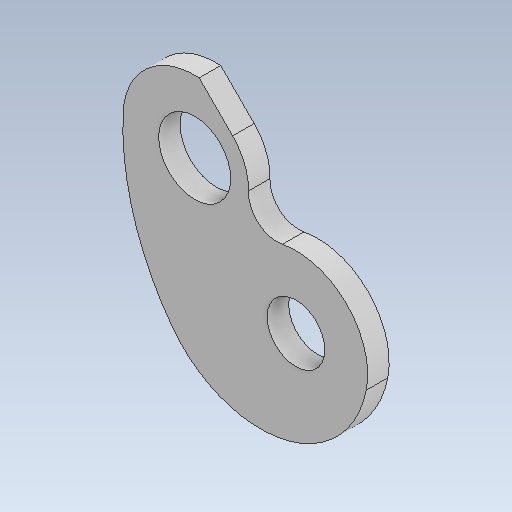
# Autodesk Inventor part: 従動節
Saved by Autodesk Inventor 2020.4 (Build 244396000, 396)
## iProperties
Created: 2021-05-01
Part Number: 従動節
Material: 一般
Document SubType Name: Modeling
Designer: happy
Density: 1 g/cm^3
Appearance: 既定
Mass: 2.14193 g
Surface Area: 19.4138 cm^2
Volume: 2.14193 cm^3
Author: happy
Autodesk Inventor part; units mm, degrees
ref_plane "YZ Plane" through (0, 0, 0) normal (1, 0, 0) x (0, 1, 0)
ref_plane "XZ Plane" through (0, 0, 0) normal (0, 1, 0) x (-1, 0, 0)
ref_plane "XY Plane" through (0, 0, 0) normal (0, 0, 1) x (1, 0, 0)
sketch "スケッチ1" plane through (0, 0, 0) normal (0, 0, 1) x (1, 0, 0)
  circle A0 centre (0, 0) radius 5.025
  circle A1 centre (0, 0) radius 10
  line L0 (0, 0) -> (14.1421, -14.1421)
  line L1 (0, 0) -> (20, 0) construction
  line L2 (0, 0) -> (14.1421, -14.1421) construction
  line L3 (-7.0711, -7.0711) -> (7.0711, -21.2132)
  line L4 (21.2132, -7.0711) -> (7.0711, 7.0711)
  arc A2 (7.0711, 7.0711) -> (-7.0711, -7.0711) centre (0, 0) ccw
  arc A3 (7.0711, -21.2132) -> (21.2132, -7.0711) centre (14.1421, -14.1421) ccw
  circle A4 centre (14.1421, -14.1421) radius 4.025
  circle A5 centre (14.1421, -14.1421) radius 13
  circle A6 centre (14.1421, -14.1421) radius 14
  line L5 (4.2426, -24.0416) -> (21.0227, -40.8217)
  line L6 (21.0227, -40.8217) -> (47.0109, -27.2119)
  line L7 (47.0109, -27.2119) -> (24.0416, -4.2426)
  arc A7 (12.0122, -27.9792) -> (10.7234, -30.5224) centre (11.784, -29.4617) ccw
  line L8 (-8.3867, -5.4464) -> (8.8712, -32.0212)
  arc A8 (10.5855, -29.4018) -> (10.585, -29.4134) centre (11.784, -29.4617) ccw
  line L9 (4.2426, -24.0416) -> (21.0227, -40.8217)
  line L10 (21.0227, -40.8217) -> (47.0109, -27.2119)
  line L11 (47.0109, -27.2119) -> (24.0416, -4.2426)
  arc A9 (8.8712, -32.0212) -> (10.7228, -30.5218) centre (9.8758, -31.3688) ccw
  arc A10 (11.5527, -27.9797) -> (10.7228, -30.5218) centre (11.784, -29.4617) ccw
  arc A11 (11.5527, -27.9797) -> (23.9469, -16.1083) centre (9.2397, -13.1591) ccw
  arc A12 (-9.9898, 0.4505) -> (9.3407, -32.4405) centre (24.9746, -1.1263) ccw
  arc A13 (21.2132, -7.0711) -> (7.0711, -21.2132) centre (14.1421, -14.1421) ccw
  arc A14 (7.4956, -0.2576) -> (12.25, -4.3228) centre (11.4932, -0.395) ccw
  circle A15 centre (0, 0) radius 7.5
  line L12 (5.3033, 5.3033) -> (0.6262, 9.9804)
  arc A16 (-3.1585, -21.9475) -> (11.5527, -27.9797) centre (9.1773, -12.8178) ccw
  point P0 (7.0711, -7.0711)
  point P1 (7.0711, 7.0711)
  point P2 (10.4941, -23.453)
  point P3 (-8.3867, -5.4464)
  point P4 (9.5568, -27.6782)
  point P5 (9.5574, -27.6666)
  point P6 (-9.9898, 0.4505)
  point P7 (10.7234, -30.5224)
  point P8 (11.5527, -27.9797)
  point P9 (9.2796, -3.7267)
  point P10 (0.6262, 9.9804)
  dimension "d0" = 10.05
  dimension "d1" = 20
  dimension "d2" = 20
  dimension "d3" = 45
  dimension "d6" = 8.05
  dimension "d7" = 26
  dimension "d8" = 1
  dimension "d9" = 1.5
  dimension "d14" = 0
  dimension "d15" = 0
  dimension "d17" = 15
  dimension "d18" = 168
  dimension "d19" = 35
  dimension "d20" = 4
  dimension "d21" = 15
  constraints: 35 point on circle, 28 end point, 22 tangent, 17 centre point, 5 coincident, 4 parallel, 2 point on line, 1 collinear, 1 equal length, 1 horizontal, 1 midpoint, 2 other
  measures "d0" diameter of A0
  measures "d1" diameter of A1
  measures "d2" distance of L0.start L0.end
  measures "d3" angle of L0 L1
  measures "d6" diameter of A4
  measures "d7" diameter of A5
  measures "d8" radial gap between concentric circles of A5 A6
  measures "d9" radius of A7
  measures "d14" distance between parallel lines of L5 L9
  measures "d15" radial gap between concentric circles of A7 A10
  measures "d17" radius of A11
  measures "d19" radius of A12
  measures "d20" radius of A14
  measures "d21" diameter of A15
extrude "押し出し1" add sketch "スケッチ1" along normal blind 3 contours A6 A15 | A6 A15 A5 L0 | L0 A5 A15 A6 | A5 A15 L0 | L0 A15 A5 | A15 A14 A6 | A6 A14 A5 A15 | A15 A5 A1 A6 | A6 A1 L12 A15 | A15 A5 A14 A1 L0 | L0 A1 A5 A15 | A6 L3 A1 | A1 A5 L3 A6 | A13 L3 A5 A1 | A1 A14 A13 | A13 A3 | L3 A6 L5 A16 L8 A1 | L3 A5 A11 A6 | A3 A11 A5 L3 | L8 A16 A12 A1 | A6 A11 A16 L5
